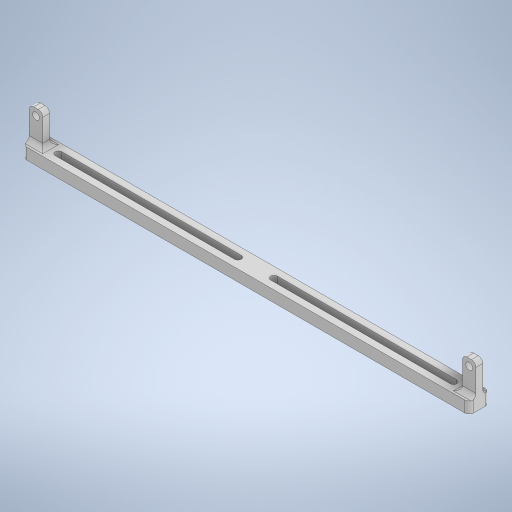
# Autodesk Inventor part: Brace_slide_v3
Saved by Autodesk Inventor 2024.3 (Build 283343000, 343)
## iProperties
Created: 2024-10-15
Part Number: Brace_slide_v3
Material: Generic
Document SubType Name: Modeling
Designer: magn1
Density: 1 g/cm^3
Appearance: Default
Author: magn1
Autodesk Inventor part; units mm, degrees
ref_plane "YZ Plane" through (0, 0, 0) normal (1, 0, 0) x (0, 1, 0)
ref_plane "XZ Plane" through (0, 0, 0) normal (0, 1, 0) x (-1, 0, 0)
ref_plane "XY Plane" through (0, 0, 0) normal (0, 0, 1) x (1, 0, 0)
sketch "Sketch1" plane through (0, 0, 0) normal (0, 1, 0) x (-1, 0, 0)
  line L0 (99.05, 4.5) -> (-99.05, 4.5)
  line L1 (-99.05, 4.5) -> (-99.05, -4.5)
  line L2 (-99.05, -4.5) -> (99.05, -4.5)
  line L3 (99.05, -4.5) -> (99.05, 4.5)
  line L4 (99.05, 4.5) -> (-99.05, -4.5) construction
  line L5 (-99.05, 4.5) -> (99.05, -4.5) construction
  line L6 (99.05, 0) -> (87.55, 0) construction
  line L7 (-99.05, 0) -> (-87.55, 0) construction
  circle A0 centre (-87.55, 0) radius 1.5
  circle A1 centre (87.55, 0) radius 1.5
  line L8 (87.55, -1.5) -> (-87.55, -1.5)
  line L9 (99.05, 4.5) -> (99.05, 12.375)
  line L10 (99.05, 4.5) -> (106.925, 4.5) construction
  line L11 (99.05, 12.375) -> (94.05, 12.375)
  line L12 (94.05, 12.375) -> (94.05, 20.375)
  line L13 (94.05, 20.375) -> (99.05, 20.375)
  line L14 (99.05, 20.375) -> (99.05, 12.375)
  line L15 (94.05, 12.375) -> (94.05, 4.5)
  line L16 (94.05, 12.375) -> (101.925, 12.375) construction
  line L17 (-99.05, 4.5) -> (-99.05, 12.375)
  line L18 (-99.05, 4.5) -> (-91.175, 4.5) construction
  line L19 (-99.05, 12.375) -> (-94.05, 12.375)
  line L20 (-94.05, 12.375) -> (-94.05, 20.375)
  line L21 (-94.05, 20.375) -> (-99.05, 20.375)
  line L22 (-99.05, 20.375) -> (-99.05, 12.375)
  line L23 (-94.05, 12.375) -> (-94.05, 4.5)
  line L24 (-94.05, 12.375) -> (-86.175, 12.375) construction
  circle A2 centre (0, 0) radius 1.5
  line L25 (0, -1.5) -> (-8, -1.5) construction
  line L26 (0, -1.5) -> (8, -1.5) construction
  circle A3 centre (8, 0) radius 1.5
  circle A4 centre (-8, 0) radius 1.5
  line L27 (96.55, 20.375) -> (96.55, 17.375) construction
  line L28 (-96.55, 20.375) -> (-96.55, 17.375) construction
  circle A5 centre (-96.55, 17.375) radius 1.5
  circle A6 centre (96.55, 17.375) radius 1.5
  line L29 (87.55, 1.5) -> (-87.55, 1.5)
  point P0 (-94.05, 4.5)
  point P1 (8, -1.5)
  point P2 (-8, -1.5)
  point P3 (8.3564, -1.4534)
  point P4 (-7.6436, -1.4608)
  point P5 (-8, 1.5)
  point P6 (8, 1.5)
  dimension "d27" = 3
  dimension "d0" = 198.1
  dimension "d1" = 9
  dimension "d2" = 11.5
  dimension "d3" = 11.5
  dimension "d4" = 3
  dimension "d5" = 3
  dimension "d8" = 7.875
  dimension "d9" = 90
  dimension "d10" = 5
  dimension "d11" = 8
  dimension "d12" = 90
  dimension "d13" = 7.875
  dimension "d14" = 90
  dimension "d15" = 5
  dimension "d16" = 8
  dimension "d17" = 90
  dimension "d28" = 8
  dimension "d29" = 8
  dimension "d30" = 3
  dimension "d31" = 3
  dimension "d32" = 1.5
  dimension "d33" = 8
  dimension "d34" = 8
  dimension "d35" = 1.5
  dimension "d36" = 3
  dimension "d37" = 3
  dimension "d38" = 3
  dimension "d39" = 3
  constraints: 60 end point, 9 horizontal, 8 perpendicular, 7 midpoint, 7 parallel, 6 centre point, 5 coincident, 4 point on circle, 4 point on line, 3 tangent, 3 vertical, 1 vertical alignment, 2 other
  measures "d0" distance of L2.end L1.end
  measures "d1" distance between parallel lines of L0 L2
  measures "d2" distance of L6.start L6.end
  measures "d3" distance of L7.start L7.end
  measures "d4" diameter of A0
  measures "d5" diameter of A1
  measures "d8" distance of L0.start L9.end
  measures "d9" angle of L10 L9
  measures "d10" distance of L12.end L13.end
  measures "d11" distance of L11.end L12.end
  measures "d12" angle of L15 L16
  measures "d13" distance of L0.end L17.end
  measures "d14" angle of L18 L17
  measures "d15" distance of L21.end L20.end
  measures "d16" distance of L20.end L19.end
  measures "d17" angle of L23 L24
  measures "d28" distance of L25.start L25.end
  measures "d29" distance of L25.start L26.end
  measures "d30" diameter of A3
  measures "d31" diameter of A4
  measures "d32" distance of A4.centre L25.end
  measures "d33" distance of A4.centre point (0, 0)
  measures "d34" distance of A3.centre point (0, 0)
  measures "d35" distance of L26.end A3.centre
  measures "d36" distance of L27.start L27.end
  measures "d37" distance of L28.start L28.end
  measures "d38" diameter of A5
  measures "d39" diameter of A6
extrude "Extrusion1" add sketch "Sketch1" along normal blind 5 contours L3 L2 L1 L0 | L29 A2 L8 A4 | L29 A3 L8 A2 | A2
sketch "Sketch4" plane through (0, 5, 0) normal (0, 1, 0) x (1, 0, 0)
  line L0 (99.05, -4.5) -> (99.05, 4.5) construction
  line L1 (99.05, 0) -> (109.05, 0) construction
  line L2 (99.05, 0) -> (96.05, 0) construction
  line L3 (99.05, -1.5) -> (93.05, -1.5)
  line L4 (93.05, -1.5) -> (93.05, 1.5)
  line L5 (93.05, 1.5) -> (99.05, 1.5)
  line L6 (99.05, 1.5) -> (99.05, -1.5)
  line L7 (99.05, -1.5) -> (93.05, 1.5) construction
  line L8 (93.05, -1.5) -> (99.05, 1.5) construction
  line L9 (-99.05, 4.5) -> (-99.05, -4.5) construction
  line L10 (-99.05, 0) -> (-93.05, 0) construction
  line L11 (-99.05, -1.5) -> (-93.05, -1.5)
  line L12 (-93.05, -1.5) -> (-93.05, 1.5)
  line L13 (-93.05, 1.5) -> (-99.05, 1.5)
  line L14 (-99.05, 1.5) -> (-99.05, -1.5)
  line L15 (-99.05, -1.5) -> (-93.05, 1.5) construction
  line L16 (-93.05, -1.5) -> (-99.05, 1.5) construction
  point P0 (0, 0)
  point P1 (-96.05, 0)
  dimension "d54" = 3
  dimension "d55" = 6
  dimension "d56" = 3
  dimension "d57" = 6
  dimension "d58" = 6
  dimension "d59" = 3
  constraints: 30 end point, 7 midpoint, 5 horizontal, 4 parallel, 2 perpendicular
  measures "d54" distance of L1.start L2.end
  measures "d55" distance of L4.end L5.end
  measures "d56" distance of L3.end L4.end
  measures "d57" distance of L10.start L10.end
  measures "d58" distance of L13.end L12.end
  measures "d59" distance of L12.end L11.end
extrude "Extrusion4" add sketch "Sketch4" along normal blind 14
sketch "Sketch5" plane through (-99.05, 5, 1.5) normal (0, 0, 1) x (1, 0, 0)
  line L0 (6, 14) -> (0, 14) construction
  line L1 (3, 14) -> (3, 11) construction
  circle A0 centre (3, 11) radius 1.5
  line L2 (198.1, 14) -> (192.1, 14) construction
  line L3 (195.1, 14) -> (195.1, 11) construction
  line L4 (195.1, 14) -> (198.1, 14) construction
  circle A1 centre (195.1, 11) radius 1.5
  point P0 (99.05, -5)
  dimension "d62" = 3
  dimension "d63" = 3
  dimension "d64" = 3
  dimension "d65" = 90
  dimension "d66" = 3
  constraints: 6 end point, 2 centre point, 2 coincident, 2 midpoint, 2 vertical, 1 horizontal, 1 perpendicular
  measures "d62" distance of L1.start L1.end
  measures "d63" diameter of A0
  measures "d64" distance of L3.start L3.end
  measures "d65" angle of L3 L4
  measures "d66" diameter of A1
extrude "Extrusion5" cut sketch "Sketch5" against normal through all
fillet "Fillet4" radius 2 4 edges at (99.05, 19, 0) (93.05, 19, 0) (-93.05, 19, 0) (-99.05, 19, 0)
fillet "Fillet5" radius 2 10 edges at (-96.05, 5, 1.5) (-96.05, 5, -1.5) (-93.05, 5, 0) (96.05, 5, 1.5) (93.05, 5, 0) (96.05, 5, -1.5) (99.05, 2.5, 4.5) (99.05, 2.5, -4.5) (-99.05, 2.5, 4.5) (-99.05, 2.5, -4.5)
body "Solid1"
